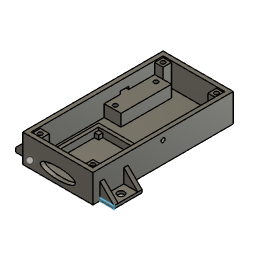
Boitier AquaTrack v2 (Autodesk Fusion 360 design; units mm, degrees)
Autodesk Fusion 360 part; units mm, degrees
note: some values were not read from the file. Chosen so that the rebuilt part matches the saved one: that a step has no effect; the layout of a text. Set by a fixed rule: which sketch regions a step uses.
sketch "Esquisse1" plane through (0, 0, 0) normal (0, 1, 0) x (1, 0, 0)
  line L0 (0, 0) -> (50, 0)
  line L1 (50, 0) -> (50, 100)
  line L2 (50, 100) -> (0, 100)
  line L3 (0, 100) -> (0, 0)
  constraint horizontal L0
  constraint vertical L1
  constraint horizontal L2
  constraint vertical L3
  constraint coincident L0.start L3.end
extrude "Extrusion1" add sketch "Esquisse1" along normal blind 3 makes body 1
sketch "Esquisse2" plane through (0, 3, 0) normal (0, 1, 0) x (-1, 0, 0)
  line L0 (0, -100) -> (0, 0)
  line L1 (0, 0) -> (-50, 0)
  line L2 (-50, 0) -> (-50, -100)
  line L3 (-50, -100) -> (0, -100)
  line L4 (-47, -97) -> (-3, -97)
  line L5 (-3, -97) -> (-3, -3)
  line L6 (-3, -3) -> (-47, -3)
  line L7 (-47, -3) -> (-47, -97)
  dimension "d3" = -3
extrude "Extrusion2" add sketch "Esquisse2" along normal blind 17 bodies 1
sketch "Esquisse3" plane through (0, 3, 0) normal (0, 1, 0) x (-1, 0, 0)
  line L0 (-47, -97) -> (-3, -97)
  line L1 (-3, -97) -> (-3, -3)
  line L2 (-3, -3) -> (-47, -3)
  line L3 (-47, -3) -> (-47, -97)
  line L4 (-11.970678, -7.104511) -> (-37.970678, -7.104511)
  line L5 (-37.970678, -7.104511) -> (-37.970678, -42.104511)
  line L6 (-37.970678, -42.104511) -> (-11.970678, -42.104511)
  line L7 (-11.970678, -42.104511) -> (-11.970678, -7.104511)
  line L8 (-9.470678, -4.604511) -> (-40.470678, -4.604511)
  line L9 (-40.470678, -4.604511) -> (-40.470678, -44.604511)
  line L10 (-40.470678, -44.604511) -> (-9.470678, -44.604511)
  line L11 (-9.470678, -44.604511) -> (-9.470678, -4.604511)
  dimension "d6" = 26
  dimension "d7" = 35
  dimension "d8" = 2.5
  constraint horizontal L4
  constraint vertical L5
  constraint horizontal L6
  constraint vertical L7
extrude "Extrusion3" add sketch "Esquisse3" along normal blind 5 contours L8 L9 L10 L11 picked at (-39.637345, -18.771177) bodies 1
sketch "Esquisse4" plane through (0, 3, 0) normal (0, 1, 0) x (-1, 0, 0)
  line L0 (-11.970678, -7.104511) -> (-37.970678, -7.104511)
  line L1 (-37.970678, -7.104511) -> (-37.970678, -42.104511)
  line L2 (-37.970678, -42.104511) -> (-11.970678, -42.104511)
  line L3 (-11.970678, -42.104511) -> (-11.970678, -7.104511)
  line L4 (-11.970678, -42.104511) -> (-14.970678, -42.104511)
  line L5 (-14.970678, -42.104511) -> (-14.970678, -39.104511)
  line L6 (-14.970678, -39.104511) -> (-11.970678, -39.104511)
  line L7 (-11.970678, -39.104511) -> (-11.970678, -42.104511)
  line L8 (-37.970678, -42.104511) -> (-34.970678, -42.104511)
  line L9 (-34.970678, -42.104511) -> (-34.970678, -39.104511)
  line L10 (-34.970678, -39.104511) -> (-37.970678, -39.104511)
  line L11 (-37.970678, -39.104511) -> (-37.970678, -42.104511)
  line L12 (-37.970678, -7.104511) -> (-34.970678, -7.104511)
  line L13 (-34.970678, -7.104511) -> (-34.970678, -10.104511)
  line L14 (-34.970678, -10.104511) -> (-37.970678, -10.104511)
  line L15 (-37.970678, -10.104511) -> (-37.970678, -7.104511)
  dimension "d11" = 3
  dimension "d12" = 3
  dimension "d13" = 3
  dimension "d14" = 3
  dimension "d15" = 3
  dimension "d16" = 3
  constraint horizontal L4
  constraint vertical L5
  constraint horizontal L6
  constraint vertical L7
  constraint horizontal L8
  constraint vertical L9
  constraint horizontal L10
  constraint vertical L11
  constraint horizontal L12
  constraint vertical L13
  constraint horizontal L14
  constraint vertical L15
extrude "Extrusion4" add sketch "Esquisse4" along normal blind 3 contours L0 L1 L12 L13 L14 L15 | L2 L3 L4 L5 L6 L7 | L1 L2 L8 L9 L10 L11 picked at (-35.970678, -9.104511) picked at (-13.970678, -41.104511) picked at (-35.970678, -40.104511) bodies 1
sketch "Esquisse5" plane through (0, 8, 0) normal (0, 1, 0) x (-1, 0, 0)
  line L0 (-11.970678, -7.104511) -> (-11.970678, -42.104511)
  line L1 (-11.970678, -42.104511) -> (-37.970678, -42.104511)
  line L2 (-37.970678, -42.104511) -> (-37.970678, -7.104511)
  line L3 (-37.970678, -7.104511) -> (-11.970678, -7.104511)
  line L4 (-9.470678, -44.604511) -> (-9.470678, -4.604511)
  line L5 (-9.470678, -4.604511) -> (-40.470678, -4.604511)
  line L6 (-40.470678, -4.604511) -> (-40.470678, -44.604511)
  line L7 (-40.470678, -44.604511) -> (-9.470678, -44.604511)
  line L8 (-34.889567, -7.104511) -> (-34.889567, -4.604511)
  line L9 (-11.970678, -7.104511) -> (-9.470678, -7.104511)
  constraint perpendicular L5 L8
  constraint perpendicular L4 L9
extrude "Extrusion5" cut sketch "Esquisse5" against normal blind 5 contours L3 L4 L5 L8 L9 picked at (-18.776974, -5.437844) bodies 1
sketch "Esquisse6" plane through (0, 3, 0) normal (0, 1, 0) x (-1, 0, 0)
  line L0 (-47, -97) -> (-3, -97)
  line L1 (-3, -97) -> (-3, -3)
  line L2 (-3, -3) -> (-47, -3)
  line L3 (-47, -3) -> (-47, -97)
  line L4 (-9.470678, -44.604511) -> (-40.470678, -44.604511)
  line L5 (-40.470678, -44.604511) -> (-40.470678, -4.604511)
  line L6 (-40.470678, -4.604511) -> (-34.889567, -4.604511)
  line L7 (-34.889567, -4.604511) -> (-34.889567, -7.104511)
  line L8 (-34.889567, -7.104511) -> (-34.970678, -7.104511)
  line L9 (-34.970678, -7.104511) -> (-34.970678, -10.104511)
  line L10 (-34.970678, -10.104511) -> (-37.970678, -10.104511)
  line L11 (-37.970678, -10.104511) -> (-37.970678, -39.104511)
  line L12 (-37.970678, -39.104511) -> (-34.970678, -39.104511)
  line L13 (-34.970678, -39.104511) -> (-34.970678, -42.104511)
  line L14 (-34.970678, -42.104511) -> (-14.970678, -42.104511)
  line L15 (-14.970678, -42.104511) -> (-14.970678, -39.104511)
  line L16 (-14.970678, -39.104511) -> (-11.970678, -39.104511)
  line L17 (-11.970678, -39.104511) -> (-11.970678, -7.104511)
  line L18 (-11.970678, -7.104511) -> (-9.470678, -7.104511)
  line L19 (-9.470678, -7.104511) -> (-9.470678, -44.604511)
  line L20 (-3, -3) -> (-9.470678, -3)
  line L21 (-9.470678, -3) -> (-9.470678, -9.5)
  line L22 (-9.470678, -9.5) -> (-3, -9.5)
  line L23 (-3, -9.5) -> (-3, -3)
  line L24 (-47, -3) -> (-41.000001, -3)
  line L25 (-41.000001, -3) -> (-41.000001, -9)
  line L26 (-41.000001, -9) -> (-47, -9)
  line L27 (-47, -9) -> (-47, -3)
  line L28 (-47, -97) -> (-41, -97)
  line L29 (-41, -97) -> (-41, -91)
  line L30 (-41, -91) -> (-47, -91)
  line L31 (-47, -91) -> (-47, -97)
  line L32 (-3, -97) -> (-9, -97)
  line L33 (-9, -97) -> (-9, -91)
  line L34 (-9, -91) -> (-3, -91)
  line L35 (-3, -91) -> (-3, -97)
  dimension "d22" = 6.5
  dimension "d23" = 6
  dimension "d24" = 6
  dimension "d25" = 6
  dimension "d26" = 6
  constraint horizontal L20
  constraint vertical L21
  constraint horizontal L22
  constraint vertical L23
  constraint coincident L1.end L2.start
  constraint horizontal L24
  constraint vertical L25
  constraint horizontal L26
  constraint vertical L27
  constraint coincident L2.end L3.start
  constraint horizontal L28
  constraint vertical L29
  constraint horizontal L30
  constraint vertical L31
  constraint coincident L0.start L3.end
  constraint horizontal L32
  constraint vertical L33
  constraint horizontal L34
  constraint vertical L35
  constraint coincident L0.end L1.start
  measures "d22" distance of L1.end L22.end
  measures "d23" distance of L0.start L28.end
  measures "d24" distance of L0.start L30.end
  measures "d25" distance of L0.end L32.end
  measures "d26" distance of L0.end L34.end
extrude "Extrusion6" add sketch "Esquisse6" along normal blind 16 contours L0 L3 L28 L29 L30 L31 | L0 L1 L32 L33 L34 L35 | L2 L3 L24 L25 L26 L27 | L1 L2 L19 L20 L21 L22 L23 picked at (-45, -93) picked at (-7, -93) picked at (-45, -5) picked at (-5.156893, -6.534837) bodies 1
sketch "Esquisse7" plane through (0, 19, 0) normal (0, 1, 0) x (-1, 0, 0)
  line L0 (-3, -91) -> (-9, -91)
  line L1 (-9, -91) -> (-9, -97)
  line L2 (-9, -97) -> (-3, -97)
  line L3 (-3, -97) -> (-3, -91)
  circle A0 centre (-6, -94) radius 1.5
  circle A1 centre (-44.000001, -94.000001) radius 1.5
  circle A2 centre (-6.25, -6.25) radius 1.5
  line L4 (-47.000001, -9) -> (-41.000001, -9)
  circle A3 centre (-44.000001, -6) radius 1.5
  dimension "d29" = 3
  dimension "d30" = 3
  dimension "d31" = 3
  dimension "d32" = 3
  constraint horizontal L4
  measures "d29" diameter of A0
  measures "d30" diameter of A1
  measures "d31" diameter of A2
  measures "d32" diameter of A3
extrude "Extrusion7" cut sketch "Esquisse7" against normal blind 15 contours A0 | A1 | A2 | A3 picked at (-5.962635, -92.938078) picked at (-43.527799, -93.927145) picked at (-7.244416, -6.324521) picked at (-44.372111, -5.734435) bodies 1
sketch "Esquisse8" plane through (0, 0, 0) normal (0, 0, 1) x (1, 0, 0)
  line L0 (0, 0) -> (50, 0)
  line L1 (50, 0) -> (50, 20)
  line L2 (50, 20) -> (0, 20)
  line L3 (0, 20) -> (0, 0)
  ellipse E0 centre (25, 7) end of major axis (37.5, 7) minor radius 4
  line L4 (12.5, 7) -> (37.5, 7) construction
  line L5 (25, 3) -> (25, 11) construction
  dimension "d35" = 25
  dimension "d36" = 8
  constraint coincident E0 L4.start
  constraint coincident E0 L4.end
  constraint coincident E0 L5.start
  constraint coincident E0 L5.end
  constraint horizontal L4
  measures "d35" distance of E0
extrude "Extrusion8" cut sketch "Esquisse8" against normal blind 3 contours E0 picked at (22.776169, 8.237259) bodies 1
sketch "Esquisse9" plane through (47, 0, 0) normal (-1, 0, 0) x (0, 0, 1)
  line L0 (-97, 19) -> (-91, 19)
  line L1 (-91, 19) -> (-91, 3)
  line L2 (-91, 3) -> (-9, 3)
  line L3 (-9, 3) -> (-9, 19)
  line L4 (-9, 19) -> (-3, 19)
  line L5 (-3, 19) -> (-3, 20)
  line L6 (-3, 20) -> (-97, 20)
  line L7 (-97, 20) -> (-97, 19)
  circle A0 centre (-50.000001, 15) radius 1.45
  dimension "d39" = 2.9
  measures "d39" diameter of A0
extrude "Extrusion9" cut sketch "Esquisse9" against normal blind 3 contours A0 picked at (-49.543059, 14.647825) bodies 1
sketch "Esquisse10" plane through (0, 3, 0) normal (0, 1, 0) x (-1, 0, 0)
  line L0 (-9, -97) -> (-9, -91)
  line L1 (-9, -91) -> (-3, -91)
  line L2 (-3, -91) -> (-3, -9.5)
  line L3 (-3, -9.5) -> (-9.470678, -9.5)
  line L4 (-9.470678, -9.5) -> (-9.470678, -44.604511)
  line L5 (-9.470678, -44.604511) -> (-40.470678, -44.604511)
  line L6 (-40.470678, -44.604511) -> (-40.470678, -4.604511)
  line L7 (-40.470678, -4.604511) -> (-34.889567, -4.604511)
  line L8 (-34.889567, -4.604511) -> (-34.889567, -7.104511)
  line L9 (-34.889567, -7.104511) -> (-34.970678, -7.104511)
  line L10 (-34.970678, -7.104511) -> (-34.970678, -10.104511)
  line L11 (-34.970678, -10.104511) -> (-37.970678, -10.104511)
  line L12 (-37.970678, -10.104511) -> (-37.970678, -39.104511)
  line L13 (-37.970678, -39.104511) -> (-34.970678, -39.104511)
  line L14 (-34.970678, -39.104511) -> (-34.970678, -42.104511)
  line L15 (-34.970678, -42.104511) -> (-14.970678, -42.104511)
  line L16 (-14.970678, -42.104511) -> (-14.970678, -39.104511)
  line L17 (-14.970678, -39.104511) -> (-11.970678, -39.104511)
  line L18 (-11.970678, -39.104511) -> (-11.970678, -7.104511)
  line L19 (-11.970678, -7.104511) -> (-9.470678, -7.104511)
  line L20 (-9.470678, -7.104511) -> (-9.470678, -3)
  line L21 (-9.470678, -3) -> (-25, -3)
  line L22 (-25, -3) -> (-41.000001, -3)
  line L23 (-41.000001, -3) -> (-41.000001, -9)
  line L24 (-41.000001, -9) -> (-47, -9)
  line L25 (-47, -9) -> (-47, -91)
  line L26 (-47, -91) -> (-41, -91)
  line L27 (-41, -91) -> (-41, -97)
  line L28 (-41, -97) -> (-9, -97)
  line L29 (-3, -91) -> (-15, -91)
  line L30 (-15, -91) -> (-15, -55.000001)
  line L31 (-15, -55.000001) -> (-3, -55.000001)
  line L32 (-3, -55.000001) -> (-3, -91)
  constraint horizontal L29
  constraint vertical L30
  constraint horizontal L31
  constraint vertical L32
  constraint coincident L1.end L2.start
extrude "Extrusion10" add sketch "Esquisse10" along normal blind 8.5 contours L1 L2 L29 L30 L31 L32 picked at (-9, -67.000001) bodies 1
sketch "Esquisse11" plane through (3, 0, 0) normal (1, 0, 0) x (0, 0, -1)
  line L0 (55.000001, 3) -> (55.000001, 11.5)
  line L1 (55.000001, 11.5) -> (91, 11.5)
  line L2 (91, 11.5) -> (91, 19)
  line L3 (91, 19) -> (97, 19)
  line L4 (97, 19) -> (97, 20)
  line L5 (97, 20) -> (3, 20)
  line L6 (3, 20) -> (3, 19)
  line L7 (3, 19) -> (9.5, 19)
  line L8 (9.5, 19) -> (9.5, 3)
  line L9 (9.5, 3) -> (55.000001, 3)
  line L10 (66.499999, 11.5) -> (72.499999, 11.5)
  line L11 (72.499999, 11.5) -> (72.499999, 13.5)
  line L12 (72.499999, 13.5) -> (66.499999, 13.5)
  line L13 (66.499999, 13.5) -> (66.499999, 11.5)
  dimension "d44" = 6
  dimension "d45" = 2
  constraint horizontal L10
  constraint vertical L11
  constraint horizontal L12
  constraint vertical L13
extrude "Extrusion11" cut sketch "Esquisse11" against normal blind 3 contours L1 L10 L11 L12 L13 picked at (68.499999, 12.833333) bodies 1
sketch "Esquisse12" plane through (0, 11.5, 0) normal (0, 1, 0) x (-1, 0, 0)
  line L0 (-3, -55.000001) -> (-15, -55.000001)
  line L1 (-15, -55.000001) -> (-15, -91)
  line L2 (-15, -91) -> (-9, -91)
  line L3 (-9, -91) -> (-3, -91)
  line L4 (-3, -91) -> (-3, -72.499999)
  line L5 (-3, -72.499999) -> (0, -72.499999)
  line L6 (0, -72.499999) -> (0, -66.499999)
  line L7 (0, -66.499999) -> (-3, -66.499999)
  line L8 (-3, -66.499999) -> (-3, -55.000001)
  circle A0 centre (-8, -58.000001) radius 1.5
  circle A1 centre (-8, -87.000001) radius 1.5
  dimension "d48" = 3
  dimension "d49" = 3
  measures "d48" diameter of A0
  measures "d49" diameter of A1
extrude "Extrusion12" cut sketch "Esquisse12" against normal blind 6 contours A0 | A1 picked at (-8.111261, -57.512537) picked at (-8.209973, -87.829758) bodies 1
sketch "Esquisse13" plane through (50, 0, 0) normal (1, 0, 0) x (0, 0, -1)
  circle A0 centre (50.000001, 15) radius 1.45
  line L0 (0, 0) -> (100, 0)
  line L1 (100, 0) -> (100, 20)
  line L2 (100, 20) -> (0, 20)
  line L3 (0, 20) -> (0, 0)
  line L4 (5, 0) -> (25, 0)
  line L5 (25, 0) -> (25, 2)
  line L6 (25, 2) -> (5, 2)
  line L7 (5, 2) -> (5, 0)
  constraint horizontal L4
  constraint vertical L5
  constraint horizontal L6
  constraint vertical L7
  constraint coincident L0 L4.start
extrude "Extrusion13" add sketch "Esquisse13" along normal blind 10 contours L0 L4 L5 L6 L7 picked at (11.666667, 1.333333) bodies 1
sketch "Esquisse14" plane through (0, 2, 0) normal (0, 1, 0) x (-1, 0, 0)
  line L0 (-50, -25) -> (-50, -5)
  line L1 (-50, -5) -> (-60, -5)
  line L2 (-60, -5) -> (-60, -25)
  line L3 (-60, -25) -> (-50, -25)
  circle A0 centre (-55, -15) radius 2.5
  dimension "d54" = 5
  measures "d54" diameter of A0
extrude "Extrusion14" cut sketch "Esquisse14" against normal blind 3 contours A0 picked at (-55.750807, -14.63843) bodies 1
sketch "Esquisse15" plane through (0, 0, -5) normal (0, 0, 1) x (1, 0, 0)
  line L0 (50, 2) -> (50, 0)
  line L1 (50, 0) -> (60, 0)
  line L2 (60, 0) -> (60, 2)
  line L3 (60, 2) -> (50, 2)
sketch "Esquisse16" plane through (0, 0, -5) normal (0, 0, 1) x (1, 0, 0)
  line L0 (50.000001, 12) -> (50.000001, 2)
  line L1 (50.000001, 2) -> (60.000001, 2)
  line L2 (50.000001, 12) -> (60.000001, 2)
  constraint vertical L0
  constraint perpendicular L0 L1
extrude "Extrusion15" add sketch "Esquisse16" against normal blind 3 bodies 1
sketch "Esquisse17" plane through (0, 0, -25) normal (0, 0, -1) x (-1, 0, 0)
  line L0 (-50, 0) -> (-50, 2)
  line L1 (-50, 2) -> (-60, 2)
  line L2 (-60, 2) -> (-60, 0)
  line L3 (-60, 0) -> (-50, 0)
  line L4 (-60, 2) -> (-50, 2)
  line L5 (-50, 2) -> (-50, 12)
  line L6 (-50, 12) -> (-60, 2)
  dimension "d59" = 10
  constraint coincident L1.end L2.start
  constraint coincident L0.end L1.start
  constraint perpendicular L4 L5
  measures "d59" distance of L0.end L5.end
extrude "Extrusion16" add sketch "Esquisse17" against normal blind 3 contours L1 L4 L5 L6 picked at (-53.333333, 5.333333) bodies 1
sketch "Esquisse18" plane through (0, 0, -5) normal (0, 0, 1) x (1, 0, 0)
sketch "Esquisse19" plane through (0, 0, 0) normal (-1, 0, 0) x (0, 0, 1)
  line L0 (-66.499999, 11.5) -> (-72.499999, 11.5)
  line L1 (-72.499999, 11.5) -> (-72.499999, 13.5)
  line L2 (-72.499999, 13.5) -> (-66.499999, 13.5)
  line L3 (-66.499999, 13.5) -> (-66.499999, 11.5)
  line L4 (-100, 0) -> (0, 0)
  line L5 (0, 0) -> (0, 20)
  line L6 (0, 20) -> (-100, 20)
  line L7 (-100, 20) -> (-100, 0)
  line L8 (-5, 0) -> (-25, 0)
  line L9 (-25, 0) -> (-25, 3)
  line L10 (-25, 3) -> (-5, 3)
  line L11 (-5, 3) -> (-5, 0)
  dimension "d62" = 20
  dimension "d63" = 3
  constraint horizontal L8
  constraint vertical L9
  constraint horizontal L10
  constraint vertical L11
  constraint coincident L4 L8.start
  measures "d62" distance of L8.start L8.end
  measures "d63" distance of L8.start L10.end
extrude "Extrusion17" add sketch "Esquisse19" along normal blind 10 contours L4 L8 L9 L10 L11 picked at (-18.333333, 2) bodies 1
sketch "Esquisse20" plane through (0, 0, -5) normal (0, 0, 1) x (1, 0, 0)
  line L0 (0, 0) -> (0, 3)
  line L1 (0, 3) -> (-10, 3)
  line L2 (-10, 3) -> (-10, 0)
  line L3 (-10, 0) -> (0, 0)
  line L4 (-10, 3) -> (0, 3)
  line L5 (0, 3) -> (0, 13)
  line L6 (0, 13) -> (-10, 3)
  constraint horizontal L4
  constraint vertical L5
  constraint coincident L1.end L2.start
extrude "Extrusion18" add sketch "Esquisse20" against normal blind 3 contours L1 L4 L5 L6 picked at (-3.333333, 6.333333) bodies 1
sketch "Esquisse21" plane through (0, 0, -25) normal (0, 0, -1) x (-1, 0, 0)
  line L0 (0, 3) -> (0, 0)
  line L1 (0, 0) -> (10, 0)
  line L2 (10, 0) -> (10, 3)
  line L3 (10, 3) -> (0, 3)
  line L4 (0, 3) -> (10, 3)
  line L5 (0, 13) -> (0, 3)
  line L6 (0, 13) -> (10, 3)
  constraint horizontal L4
  constraint vertical L5
  constraint coincident L0.start L3.end
  constraint coincident L2.end L3.start
extrude "Extrusion19" add sketch "Esquisse21" against normal blind 3 contours L3 L4 L5 L6 picked at (3.333333, 6.333333) bodies 1
sketch "Esquisse22" plane through (0, 3, 0) normal (0, 1, 0) x (-1, 0, 0)
  line L0 (0, -22) -> (10, -22)
  line L1 (10, -22) -> (10, -8)
  line L2 (10, -8) -> (0, -8)
  line L3 (0, -8) -> (0, -22)
  circle A0 centre (5, -15) radius 2.5
  dimension "d71" = 5
  measures "d71" diameter of A0
extrude "Extrusion20" cut sketch "Esquisse22" against normal blind 3 contours A0 picked at (5.580754, -14.754371) bodies 1
extrude "Extrusion21" cut 1 faces at (11.970678, 5.666667, -17.771177) along direction (-1, 0, 0) blind 0.5 on bodies 1 bodies 1
extrude "Extrusion22" add 1 faces at (9.470678, 4.666667, -32.903007) along direction (-1, 0, 0) blind 0.5 on bodies 1 bodies 1
extrude "Extrusion23" cut 1 faces at (37.970678, 4, -19.771177) along direction (1, 0, 0) blind 0.5 on bodies 1 bodies 1
extrude "Extrusion24" add 1 faces at (40.470678, 6.333333, -17.937844) along direction (1, 0, 0) blind 0.5 on bodies 1 bodies 1
extrude "Extrusion25" add 1 faces at (21.637345, 4, -42.104511) along direction (0, 0, 1) blind 0.5 on bodies 1 bodies 1
extrude "Extrusion26" cut 1 faces at (30.304011, 4.666667, -44.604511) along direction (0, 0, 1) blind 0.2 on bodies 1 bodies 1
extrude "Extrusion27" add 2 faces at (36.137345, 4, -39.104511) (13.804011, 4, -39.104511) along direction (0, 0, 1) blind 0.2 on bodies 1 bodies 1
sketch "Esquisse23" plane through (47, 0, 0) normal (-1, 0, 0) x (0, 0, 1)
  circle A0 centre (-50.000001, 15) radius 1.45
  line L0 (-97, 19) -> (-91, 19)
  line L1 (-91, 19) -> (-91, 3)
  line L2 (-91, 3) -> (-9, 3)
  line L3 (-9, 3) -> (-9, 19)
  line L4 (-9, 19) -> (-3, 19)
  line L5 (-3, 19) -> (-3, 20)
  line L6 (-3, 20) -> (-97, 20)
  line L7 (-97, 20) -> (-97, 19)
  line L8 (-48.899999, 16.2) -> (-51.299999, 13.8)
extrude "Extrusion28" add sketch "Esquisse23" against normal blind 3 contours A0 L8 | A0 L8 picked at (-49.614439, 14.203001) picked at (-50.529185, 15.274893) bodies 1
sketch "Esquisse24" plane through (47, 0, 0) normal (-1, 0, 0) x (0, 0, 1)
  line L0 (-97, 19) -> (-91, 19)
  line L1 (-91, 19) -> (-91, 3)
  line L2 (-91, 3) -> (-9, 3)
  line L3 (-9, 3) -> (-9, 19)
  line L4 (-9, 19) -> (-3, 19)
  line L5 (-3, 19) -> (-3, 20)
  line L6 (-3, 20) -> (-97, 20)
  line L7 (-97, 20) -> (-97, 19)
  circle A0 centre (-50.000001, 12) radius 3
extrude "Extrusion29" cut sketch "Esquisse24" against normal blind 3 contours A0 picked at (-49.266949, 12.090663) bodies 1
sketch "Esquisse25" plane through (0, 0, -3) normal (0, 0, -1) x (-1, 0, 0)
  line L0 (-9.470678, 3) -> (-9.470678, 19)
  line L1 (-9.470678, 19) -> (-3, 19)
  line L2 (-3, 19) -> (-3, 20)
  line L3 (-3, 20) -> (-47, 20)
  line L4 (-47, 20) -> (-47, 19)
  line L5 (-47, 19) -> (-41.000001, 19)
  line L6 (-41.000001, 19) -> (-41.000001, 3)
  line L7 (-41.000001, 3) -> (-25, 3)
  line L8 (-25, 3) -> (-9.470678, 3)
  line L9 (-12, 3) -> (-39.500001, 3)
  line L10 (-39.500001, 3) -> (-39.500001, 13.5)
  line L11 (-39.500001, 13.5) -> (-12, 13.5)
  line L12 (-12, 13.5) -> (-12, 3)
  constraint horizontal L9
  constraint vertical L10
  constraint horizontal L11
  constraint vertical L12
  constraint coincident L8 L9.start
extrude "Extrusion30" cut sketch "Esquisse25" against normal blind 3 contours L7 L8 L9 L10 L11 L12 picked at (-25.5, 10) bodies 1
sketch "Esquisse26" plane through (11.470678, 0, 0) normal (1, 0, 0) x (0, 0, -1)
  line L0 (38.904511, 6) -> (41.604511, 6)
  line L1 (41.604511, 6) -> (41.604511, 8)
  line L2 (41.604511, 8) -> (7.104511, 8)
  line L3 (7.104511, 8) -> (7.104511, 3)
  line L4 (7.104511, 3) -> (38.904511, 3)
  line L5 (38.904511, 3) -> (38.904511, 6)
extrude "Extrusion31" add 1 faces at (38.943641, 6.333333, -4.604511) along direction (0, 0, 1) blind 1.605 on bodies 1 bodies 1
extrude "Extrusion32" add 1 faces at (10.804011, 6.333333, -7.104511) along direction (0, 0, 1) blind 4.105 on bodies 1 bodies 1
extrude "Extrusion33" cut 1 faces at (12, 10, -2) along direction (-1, 0, 0) blind 0.529 on bodies 1 bodies 1
extrude "Extrusion34" add 1 faces at (36.426378, 4.666667, -2.999511) along direction (0, 0, 1) blind 3 on bodies 1 bodies 1
extrude "Extrusion35" [no effect]
extrude "Extrusion36" cut 1 faces at (36.426378, 4.666667, 0.000489) along direction (0, 0, -1) blind 4.1 on bodies 1 bodies 1
extrude "Extrusion37" add 1 faces at (36.426378, 4.666667, -4.099511) along direction (0, 0, 1) blind 4.1 on bodies 1 bodies 1
extrude "Extrusion38" cut 4 faces at (6.037365, 19, -96.498602) (43.962635, 19, -91.501399) (43.962635, 19, -3.501398) (6.202861, 19, -3.584731) along direction (0, -1, 0) blind 1.5 on bodies 1 bodies 1
sketch "Esquisse27" plane through (0, 17.5, 0) normal (0, 1, 0) x (-1, 0, 0)
sketch "Esquisse28" plane through (0, 20, 0) normal (0, 1, 0) x (-1, 0, 0)
  line L0 (-47, -97) -> (-47, -3)
  line L1 (-47, -3) -> (-3, -3)
  line L2 (-3, -3) -> (-3, -97)
  line L3 (-3, -97) -> (-47, -97)
  line L4 (-50, -100) -> (0, -100)
  line L5 (0, -100) -> (0, 0)
  line L6 (0, 0) -> (-50, 0)
  line L7 (-50, 0) -> (-50, -100)
  line L8 (0, 0) -> (-50, 0)
  line L9 (-50, 0) -> (-50, -100)
  line L10 (-50, -100) -> (0, -100)
  line L11 (0, -100) -> (0, 0)
  constraint horizontal L8
  constraint vertical L9
  constraint horizontal L10
  constraint vertical L11
  constraint coincident L4.start L7.end
  constraint coincident L5.end L6.start
extrude "Extrusion1'" add sketch "Esquisse28" along normal blind 5 separate body makes body 2 in component "Couvercle (1)"
extrude "Extrusion2'" add 4 faces at (6.037365, 17.5, -96.498602) (43.962635, 17.5, -91.501399) (43.962635, 17.5, -3.501398) (6.202861, 17.5, -3.584731) along direction (0, 1, 0) blind 14 on bodies 1 bodies 2 in component "Couvercle (1)"
extrude "Extrusion3'" cut 4 faces at (6.202861, 31.5, -3.584731) (43.962635, 31.5, -3.501398) (43.962635, 31.5, -91.501399) (6.037365, 31.5, -96.498602) along direction (0, -1, 0) blind 6.5 on bodies 2 bodies 2 in component "Couvercle (1)"
extrude "Extrusion4'" cut 1 faces at (1, 25, -36.5) along direction (0, -1, 0) blind 4 on bodies 2 bodies 2 in component "Couvercle (1)"
extrude "Extrusion5'" add 1 faces at (1, 21, -36.5) along direction (0, 1, 0) blind 0.5 on bodies 2 bodies 2 in component "Couvercle (1)"
extrude "Extrusion6'" cut 4 faces at (6.202861, 17.5, -3.584731) (6.037365, 17.5, -96.498602) (43.962635, 17.5, -91.501399) (43.962635, 17.5, -3.501398) along direction (0, 1, 0) blind 1 on bodies 2 bodies 2 in component "Couvercle (1)"
sketch "Esquisse29" plane through (0, 21.5, 0) normal (0, 1, 0) x (-1, 0, 0)
  circle A0 centre (-44.000001, -94.000001) radius 1.5
  circle A1 centre (-6.25, -6.25) radius 1.5
  circle A2 centre (-44.000001, -6) radius 1.5
  circle A3 centre (-6, -94) radius 1.5
  line L0 (-3, -9.5) -> (-3, -91)
  line L1 (-3, -91) -> (-9, -91)
  line L2 (-9, -91) -> (-9, -97)
  line L3 (-9, -97) -> (-41, -97)
  line L4 (-41, -97) -> (-41, -91)
  line L5 (-41, -91) -> (-47, -91)
  line L6 (-47, -91) -> (-47, -9)
  line L7 (-47, -9) -> (-41.000001, -9)
  line L8 (-41.000001, -9) -> (-41.000001, -3)
  line L9 (-41.000001, -3) -> (-9.470678, -3)
  line L10 (-9.470678, -3) -> (-9.470678, -9.5)
  line L11 (-9.470678, -9.5) -> (-3, -9.5)
  line L12 (0, -100) -> (0, 0)
  line L13 (0, 0) -> (-50, 0)
  line L14 (-50, 0) -> (-50, -100)
  line L15 (-50, -100) -> (0, -100)
extrude "Extrusion7'" add sketch "Esquisse29" against normal blind 3 contours L0 L1 L2 L3 L4 L5 L6 L7 L8 L9 L10 L11 picked at (-19.823559, -63.833333) bodies 2 in component "Couvercle (1)"
sketch "Esquisse30" plane through (0, 18.5, 0) normal (0, -1, 0) x (1, 0, 0)
extrude "Extrusion39" add 1 faces at (39.500001, 9.833333, -1) along direction (-1, 0, 0) blind 4.61 on bodies 1 bodies 1
extrude "Extrusion40" add 1 faces at (11.471, 10, -2) along direction (1, 0, 0) blind 3 on bodies 1 bodies 1
extrude "Extrusion41" cut 1 faces at (34.889567, 6.333333, -3.734511) along direction (1, 0, 0) blind 0.081 on bodies 1 bodies 1
extrude "Extrusion42" add 1 faces at (34.970678, 4, -8.104511) along direction (-1, 0, 0) blind 0.081 on bodies 1 bodies 1
extrude "Extrusion43" add 1 faces at (34.970567, 4.666667, -2.366504) along direction (-1, 0, 0) blind 0.081 on bodies 1 bodies 1
extrude "Extrusion44" add 1 faces at (38.110452, 8, -4.36817) along direction (0, 1, 0) blind 1 on bodies 1 bodies 1
extrude "Extrusion45" cut 1 faces at (34.889567, 7, -3.734511) along direction (1, 0, 0) blind 6 on bodies 1 bodies 1
extrude "Extrusion46" add 1 faces at (36.889856, 9, -2) along direction (0, -1, 0) blind 6 on bodies 1 bodies 1
extrude "Extrusion47" add 1 faces at (40.889567, 7, -4.734674) along direction (-1, 0, 0) blind 6 on bodies 1 bodies 1
extrude "Extrusion48" add 1 faces at (34.889567, 7, -4.734674) along direction (-1, 0, 0) blind 23.419 on bodies 1 bodies 1
sketch "Esquisse31" plane through (0, 9, 0) normal (0, 1, 0) x (-1, 0, 0)
  line L0 (-14.471, -3) -> (-34.890001, -3)
  line L1 (-34.890001, -3) -> (-40.970678, -3)
  line L2 (-40.970678, -3) -> (-40.970678, -44.404511)
  line L3 (-40.970678, -44.404511) -> (-8.970678, -44.404511)
  line L4 (-8.970678, -44.404511) -> (-8.970678, -9.5)
  line L5 (-8.970678, -9.5) -> (-9.470678, -9.5)
  line L6 (-9.470678, -9.5) -> (-9.470678, -3)
  line L7 (-9.470678, -3) -> (-14.471, -3)
  line L8 (-38.470678, -7.104511) -> (-11.470678, -7.104511)
  line L9 (-11.470678, -7.104511) -> (-11.470678, -41.604511)
  line L10 (-11.470678, -41.604511) -> (-38.470678, -41.604511)
  line L11 (-38.470678, -41.604511) -> (-38.470678, -7.104511)
  line L12 (-14.5, -3) -> (-14.5, -7.104511)
  line L13 (-34.890001, -3) -> (-34.890001, -7.104511)
  constraint coincident L0 L12.start
  constraint perpendicular L8 L12
  constraint perpendicular L8 L13
extrude "Extrusion49" cut sketch "Esquisse31" against normal blind 6 contours L0 L8 L12 L13 picked at (-21.296667, -5.73634) bodies 1
extrude "Extrusion50" add 1 faces at (14.970678, 4, -40.704511) along direction (1, 0, 0) blind 20 on bodies 1 bodies 1
sketch "Esquisse32" plane through (0, 6, 0) normal (0, 1, 0) x (-1, 0, 0)
  line L0 (-38.470678, -41.604511) -> (-11.470678, -41.604511)
  line L1 (-11.470678, -41.604511) -> (-11.470678, -38.904511)
  line L2 (-11.470678, -38.904511) -> (-38.470678, -38.904511)
  line L3 (-38.470678, -38.904511) -> (-38.470678, -41.604511)
  line L4 (-11.470678, -38.904511) -> (-14.470678, -38.904511)
  line L5 (-14.470678, -38.904511) -> (-14.470678, -41.604511)
  line L6 (-14.470678, -41.604511) -> (-11.470678, -41.604511)
  line L7 (-11.470678, -41.604511) -> (-11.470678, -38.904511)
  line L8 (-14.470678, -38.904511) -> (-17.470678, -38.904511)
  line L9 (-17.470678, -38.904511) -> (-17.470678, -41.599999)
  line L10 (-17.470678, -41.599999) -> (-14.470678, -41.599999)
  line L11 (-14.470678, -41.599999) -> (-14.470678, -38.904511)
  line L12 (-17.470678, -38.904511) -> (-20.470678, -38.904511)
  line L13 (-20.470678, -38.904511) -> (-20.470678, -41.599999)
  line L14 (-20.470678, -41.599999) -> (-17.470678, -41.599999)
  line L15 (-17.470678, -41.599999) -> (-17.470678, -38.904511)
  line L16 (-20.470678, -38.904511) -> (-23.470678, -38.904511)
  line L17 (-23.470678, -38.904511) -> (-23.470678, -41.604511)
  line L18 (-23.470678, -41.604511) -> (-20.470678, -41.604511)
  line L19 (-20.470678, -41.604511) -> (-20.470678, -38.904511)
  line L20 (-23.470678, -38.904511) -> (-26.470678, -38.904511)
  line L21 (-26.470678, -38.904511) -> (-26.470678, -41.608124)
  line L22 (-26.470678, -41.608124) -> (-23.470678, -41.608124)
  line L23 (-23.470678, -41.608124) -> (-23.470678, -38.904511)
  line L24 (-26.470678, -38.904511) -> (-29.470678, -38.904511)
  line L25 (-29.470678, -38.904511) -> (-29.470678, -41.604511)
  line L26 (-29.470678, -41.604511) -> (-26.470678, -41.604511)
  line L27 (-26.470678, -41.604511) -> (-26.470678, -38.904511)
  line L28 (-29.470678, -38.904511) -> (-32.470678, -38.904511)
  line L29 (-32.470678, -38.904511) -> (-32.470678, -41.604511)
  line L30 (-32.470678, -41.604511) -> (-29.470678, -41.604511)
  line L31 (-29.470678, -41.604511) -> (-29.470678, -38.904511)
  line L32 (-32.470678, -38.904511) -> (-35.470678, -38.904511)
  line L33 (-35.470678, -38.904511) -> (-35.470678, -41.604511)
  line L34 (-35.470678, -41.604511) -> (-32.470678, -41.604511)
  line L35 (-32.470678, -41.604511) -> (-32.470678, -38.904511)
  dimension "d157" = 3
  dimension "d158" = 3
  dimension "d159" = 3
  dimension "d160" = 3
  dimension "d161" = 3
  dimension "d162" = 3
  dimension "d163" = 3
  dimension "d164" = 3
  constraint horizontal L4
  constraint vertical L5
  constraint horizontal L6
  constraint vertical L7
  constraint horizontal L8
  constraint vertical L9
  constraint horizontal L10
  constraint vertical L11
  constraint horizontal L12
  constraint vertical L13
  constraint horizontal L14
  constraint vertical L15
  constraint horizontal L16
  constraint vertical L17
  constraint horizontal L18
  constraint vertical L19
  constraint horizontal L20
  constraint vertical L21
  constraint horizontal L22
  constraint vertical L23
  constraint horizontal L24
  constraint vertical L25
  constraint horizontal L26
  constraint vertical L27
  constraint horizontal L28
  constraint vertical L29
  constraint horizontal L30
  constraint vertical L31
  constraint horizontal L32
  constraint vertical L33
  constraint horizontal L34
  constraint vertical L35
extrude "Extrusion51" cut sketch "Esquisse32" against normal blind 3 contours L2 L5 L8 L9 L10 L11 L15 picked at (-15.470678, -40.701503) bodies 1
sketch "Esquisse33" plane through (0, 6, 0) normal (0, 1, 0) x (-1, 0, 0)
  line L0 (-14.470678, -38.904511) -> (-14.470678, -41.599999)
  line L1 (-14.470678, -41.599999) -> (-17.470678, -41.599999)
  line L2 (-17.470678, -41.599999) -> (-17.470678, -38.904511)
  line L3 (-17.470678, -38.904511) -> (-38.470678, -38.904511)
  line L4 (-38.470678, -38.904511) -> (-38.470678, -41.604511)
  line L5 (-38.470678, -41.604511) -> (-11.470678, -41.604511)
  line L6 (-11.470678, -41.604511) -> (-11.470678, -38.904511)
  line L7 (-11.470678, -38.904511) -> (-14.470678, -38.904511)
  line L8 (-17.470678, -38.904511) -> (-20.470678, -38.904511)
  line L9 (-20.470678, -38.904511) -> (-20.470678, -41.604511)
  line L10 (-20.470678, -41.604511) -> (-17.470678, -41.604511)
  line L11 (-17.470678, -41.604511) -> (-17.470678, -38.904511)
  line L12 (-20.470678, -38.904511) -> (-23.470678, -38.904511)
  line L13 (-23.470678, -38.904511) -> (-23.470678, -41.604511)
  line L14 (-23.470678, -41.604511) -> (-20.470678, -41.604511)
  line L15 (-20.470678, -41.604511) -> (-20.470678, -38.904511)
  line L16 (-38.470678, -38.904511) -> (-35.470678, -38.904511)
  line L17 (-35.470678, -38.904511) -> (-35.470678, -41.604511)
  line L18 (-35.470678, -41.604511) -> (-38.470678, -41.604511)
  line L19 (-38.470678, -41.604511) -> (-38.470678, -38.904511)
  line L20 (-35.470678, -38.904511) -> (-32.470678, -38.904511)
  line L21 (-32.470678, -38.904511) -> (-32.470678, -41.604511)
  line L22 (-32.470678, -41.604511) -> (-35.470678, -41.604511)
  line L23 (-35.470678, -41.604511) -> (-35.470678, -38.904511)
  dimension "d167" = 3
  dimension "d168" = 3
  dimension "d169" = 3
  dimension "d170" = 3
  constraint horizontal L8
  constraint vertical L9
  constraint horizontal L10
  constraint vertical L11
  constraint horizontal L12
  constraint vertical L13
  constraint horizontal L14
  constraint vertical L15
  constraint horizontal L16
  constraint vertical L17
  constraint horizontal L18
  constraint vertical L19
  constraint horizontal L20
  constraint vertical L21
  constraint horizontal L22
  constraint vertical L23
extrude "Extrusion52" cut sketch "Esquisse33" against normal blind 3 contours L3 L5 L17 L20 L21 L22 L23 picked at (-34.470678, -40.704511) bodies 1
extrude "Extrusion53" cut 1 faces at (16.470678, 5, -41.599999) along direction (0, 0, -1) blind 0.005 on bodies 1 bodies 1
delete_face "DeleteFace1" 1 faces at (16.470678, 5, -41.604999) on bodies 1
extrude "Extrusion54" add 1 faces at (15.470678, 6, -43.471177) along direction (0, -1, 0) blind 3 on bodies 1 bodies 1
sketch "Esquisse34" plane through (50, 0, 0) normal (1, 0, 0) x (0, 0, -1)
  circle A0 centre (50.000001, 12) radius 3
  line L0 (25, 12) -> (25, 0)
  line L1 (25, 0) -> (100, 0)
  line L2 (100, 0) -> (100, 20)
  line L3 (100, 20) -> (0, 20)
  line L4 (0, 20) -> (0, 0)
  line L5 (0, 0) -> (5, 0)
  line L6 (5, 0) -> (5, 12)
  line L7 (5, 12) -> (8, 12)
  line L8 (8, 12) -> (8, 2)
  line L9 (8, 2) -> (22, 2)
  line L10 (22, 2) -> (22, 12)
  line L11 (22, 12) -> (25, 12)
  circle A1 centre (49.96472, 12) radius 3.25
  dimension "d177" = 6.5
  measures "d177" diameter of A1
extrude "Extrusion55" cut sketch "Esquisse34" against normal blind 3 contours A1 picked at (46.881212, 11.370177) bodies 1
sketch "Esquisse35" plane through (0, 11.5, 0) normal (0, 1, 0) x (-1, 0, 0)
  circle A0 centre (-8, -58.000001) radius 1.5
  circle A1 centre (-8, -87.000001) radius 1.5
  line L0 (-3, -55.000001) -> (-15, -55.000001)
  line L1 (-15, -55.000001) -> (-15, -91)
  line L2 (-15, -91) -> (-9, -91)
  line L3 (-9, -91) -> (-3, -91)
  line L4 (-3, -91) -> (-3, -72.499999)
  line L5 (-3, -72.499999) -> (0, -72.499999)
  line L6 (0, -72.499999) -> (0, -66.499999)
  line L7 (0, -66.499999) -> (-3, -66.499999)
  line L8 (-3, -66.499999) -> (-3, -55.000001)
  line L9 (-15, -55.000001) -> (-3, -55.000001)
  line L10 (-3, -55.000001) -> (-3, -91)
  line L11 (-3, -91) -> (-15, -91)
  line L12 (-15, -91) -> (-15, -55.000001)
  circle A2 centre (-8, -87.000001) radius 1.5
  circle A3 centre (-8, -58.000001) radius 1.5
  constraint horizontal L9
  constraint vertical L10
  constraint horizontal L11
  constraint vertical L12
  constraint coincident L3.end L4.start
  constraint tangent A1 A2
  constraint tangent A0 A3
extrude "Extrusion1''" add sketch "Esquisse35" along normal blind 1 separate body contours L0 L1 L2 L3 L4 L8 L9 L10 L11 L12 picked at (-6.956823, -72.5) makes body 3 in component "Barre de maintien"
extrude "Extrusion2''" add 1 faces at (6.956823, 12.5, -72.5) along direction (0, 1, 0) blind 1 on bodies 3 bodies 3 in component "Barre de maintien"
sketch "Esquisse1 (2)" plane through (0, 11.5, 0) normal (0, -1, 0) x (1, 0, 0) in component "Barre de maintien"
  circle A0 centre (8, -87.000001) radius 1.5
  circle A1 centre (8, -58.000001) radius 1.5
  line L0 (3, -91) -> (15, -91)
  line L1 (15, -91) -> (15, -55.000001)
  line L2 (15, -55.000001) -> (3, -55.000001)
  line L3 (3, -55.000001) -> (3, -91)
  line L4 (3, -62.270904) -> (15, -62.270904)
  line L5 (15, -62.270904) -> (15, -83.000001)
  line L6 (15, -83.000001) -> (3, -83.000001)
  line L7 (3, -83.000001) -> (3, -62.270904)
  constraint horizontal L4
  constraint vertical L5
  constraint horizontal L6
  constraint vertical L7
extrude "Extrusion3''" cut sketch "Esquisse1 (2)" against normal blind 0.5 contours L1 L3 L4 L5 L6 L7 picked at (7, -76.090302) bodies 3 in component "Barre de maintien"
sketch "Esquisse1 (3)" plane through (0, 21.5, 0) normal (0, 1, 0) x (-1, 0, 0) in component "Couvercle (1)"
  circle A0 centre (-44.000001, -94.000001) radius 1.5
  circle A1 centre (-6.25, -6.25) radius 1.5
  circle A2 centre (-44.000001, -6) radius 1.5
  circle A3 centre (-6, -94) radius 1.5
  line L0 (0, -100) -> (0, 0)
  line L1 (0, 0) -> (-50, 0)
  line L2 (-50, 0) -> (-50, -100)
  line L3 (-50, -100) -> (0, -100)
  line L4 (-10, -90) -> (-10, -10) construction
  line L5 (-10, -10) -> (-40, -10) construction
  line L6 (-40, -10) -> (-40, -90) construction
  line L7 (-40, -90) -> (-10, -90) construction
  dimension "d186" = 6
  text T0 "AquaTrack\nby Dji\nVersion 2" font "Arial Black" height 6 align centre top in box 80 x 30 at (-10, -90) x (0, 1) y (-1, 0) spacing 1 kerned
extrude "Extrusion8'" cut sketch "Esquisse1 (3)" against normal blind 0.5 text T0 bodies 2 in component "Couvercle (1)"
extrude "Extrusion4''" add 1 faces at (13.033193, 13.5, -77.326581) along direction (0, 1, 0) blind 1 on bodies 3 bodies 3 in component "Barre de maintien"
extrude "Extrusion5''" cut 1 faces at (7, 12, -76.090302) along direction (0, 1, 0) blind 0.25 on bodies 3 bodies 3 in component "Barre de maintien"
sketch "Esquisse1 (4)" plane through (0, 20, 0) normal (0, 1, 0) x (-1, 0, 0) in component "Couvercle"
  line L0 (-47, -97) -> (-47, -3)
  line L1 (-47, -3) -> (-3, -3)
  line L2 (-3, -3) -> (-3, -97)
  line L3 (-3, -97) -> (-47, -97)
  line L4 (-50, -100) -> (0, -100)
  line L5 (0, -100) -> (0, 0)
  line L6 (0, 0) -> (-50, 0)
  line L7 (-50, 0) -> (-50, -100)
  line L8 (0, 0) -> (-50, 0)
  line L9 (-50, 0) -> (-50, -100)
  line L10 (-50, -100) -> (0, -100)
  line L11 (0, -100) -> (0, 0)
  constraint horizontal L8
  constraint vertical L9
  constraint horizontal L10
  constraint vertical L11
  constraint coincident L4.start L7.end
  constraint coincident L5.end L6.start
extrude "Extrusion1'''" [suppressed] in component "Couvercle"
sketch "Esquisse2 (2)" plane through (0, 20, 0) normal (0, -1, 0) x (1, 0, 0) in component "Couvercle"
  line L0 (0, 0) -> (0, -100)
  line L1 (0, -100) -> (50, -100)
  line L2 (50, -100) -> (50, 0)
  line L3 (50, 0) -> (0, 0)
  line L4 (3.4, -96.6) -> (46.6, -96.6)
  line L5 (46.6, -96.6) -> (46.6, -3.4)
  line L6 (46.6, -3.4) -> (3.4, -3.4)
  line L7 (3.4, -3.4) -> (3.4, -96.6)
  dimension "d113" = -3.4
extrude "Extrusion2'''" [suppressed] in component "Couvercle"
extrude "Extrusion3'''" [suppressed] in component "Couvercle"
component "Couvercle (1)" placed x (1, 0, 0) y (0, 1, 0) z (0, 0, 1) at (0, 0, 0)
component "Barre de maintien" placed x (1, 0, 0) y (0, 1, 0) z (0, 0, 1) at (0, 0, 0)
named bodies: "Boitier"
